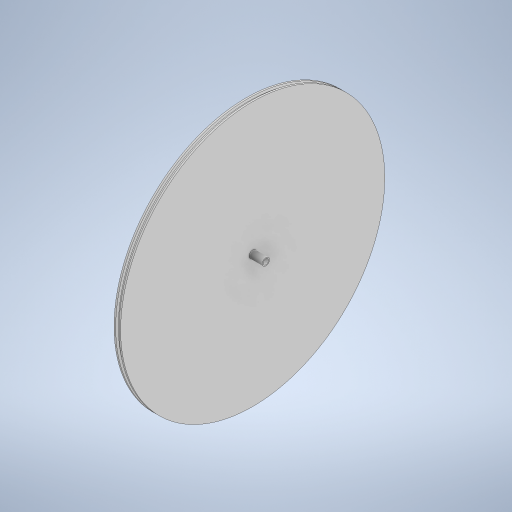
# Autodesk Inventor part: Шкив 80
Saved by Autodesk Inventor 2023 (Build 270158000, 158)
## iProperties
Created: 2022-05-01
Part Number: Шкив 80
Material: Типовые
Document SubType Name: Modeling
Designer: User
Density: 1 g/cm^3
Appearance: По умолчанию
Author: User
Autodesk Inventor part; units mm, degrees
ref_plane "YZ Plane" through (0, 0, 0) normal (1, 0, 0) x (0, 1, 0)
ref_plane "XZ Plane" through (0, 0, 0) normal (0, 1, 0) x (-1, 0, 0)
ref_plane "XY Plane" through (0, 0, 0) normal (0, 0, 1) x (1, 0, 0)
sketch "Эскиз1" plane through (0, 0, 0) normal (0, 1, 0) x (-1, 0, 0)
  line L0 (0, 0) -> (20, 0)
  line L1 (20, 0) -> (20, 400)
  line L2 (20, 400) -> (0, 400)
  line L3 (0, 400) -> (0, 0)
  line L4 (20, 400) -> (13, 400)
  line L5 (13, 400) -> (13, 394)
  line L6 (13, 394) -> (7, 394)
  line L7 (7, 394) -> (7, 400)
  dimension "d0" = 20
  dimension "d1" = 400
  dimension "d2" = 7
  dimension "d3" = 6
  dimension "d4" = 6
  constraints: 16 end point, 6 perpendicular, 2 point on line, 1 horizontal
  measures "d0" distance of L0.start L0.end
  measures "d1" distance of L0.end L1.end
  measures "d2" distance of L1.end L4.end
  measures "d3" distance of L4.end L5.end
  measures "d4" distance of L5.end L6.end
revolve "Вращение1" add sketch "Эскиз1" angle 360 about axis through (0, 0, 0) along (-1, 0, 0) contours L3 L2 L7 L6 L5 L1 L0
sketch "Эскиз2" plane through (0, 0, 0) normal (1, 0, 0) x (0, 0, -1)
  circle A0 centre (0, 0) radius 11
  dimension "d6" = 22
  constraints: 1 centre point, 1 coincident
  measures "d6" diameter of A0
extrude "Выдавливание1" add sketch "Эскиз2" along normal blind 40
sketch "Эскиз3" plane through (40, 0, 0) normal (1, 0, 0) x (0, 0, -1)
  circle A0 centre (0, 0) radius 8
  dimension "d9" = 16
  constraints: 1 centre point, 1 coincident
  measures "d9" diameter of A0
extrude "Выдавливание2" cut sketch "Эскиз3" against normal blind 88.25
chamfer "Фаска1" distance 2 distance2 6 1 edges at (-13, 0, -400) measured on face at (-13.5, 0, -400)
chamfer "Фаска2" distance 6 distance2 2 1 edges at (-7, 0, -400) measured on face at (-7, 0, -399.5)
